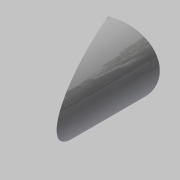
# Autodesk Inventor part: A1-19037-200-01 Trunk shell
Saved by Autodesk Inventor 2017.3 (Build 213257000, 257)
## iProperties
Created: 2019-08-22
Part Number: A1-19037-200-01 Trunk shell
Material: Steel, Mild
Document SubType Name: Sheet Metal
Designer: GVD
Density: 7.85 g/cm^3
Appearance: Steel
Project: A1-19037--CNUL Albian CST laterals
Mass: 348967 g
Surface Area: 25371.3 cm^2
Volume: 44454.4 cm^3
Description: 112 5/16" x 68 15/32" x 1 1/2" PLATE, A516 Gr.70N, ROLLED TO 37 1/4" OD
Flat Pattern Width: 131.612 cm
Flat Pattern Length: 134.186 cm
Flat Pattern Area: 17660.5 cm^2
Sheet Metal Rule: Default
Sheet Metal Width: 51.816 in
Sheet Metal Length: 52.829 in
Sheet Metal Area: 2737.386 in^2
Constructed By: Graeme_Van_Dongen
Project Name: CST laterals
Author: GVD
Autodesk Inventor part; units mm, degrees
ref_plane "YZ Plane" through (0, 0, 0) normal (1, 0, 0) x (0, 1, 0)
ref_plane "XZ Plane" through (0, 0, 0) normal (0, 1, 0) x (-1, 0, 0)
ref_plane "XY Plane" through (0, 0, 0) normal (0, 0, 1) x (1, 0, 0)
sketch "Sketch1" plane through (0, 0, 0) normal (0, 0, 1) x (1, 0, 0)
  circle A0 centre (0, 0) radius 434.975
  circle A1 centre (0, 0) radius 473.075
  circle A2 centre (0, 0) radius 436.5625
  dimension "d0" = 869.95
  dimension "d1" = 946.15
  dimension "d10" = 873.125
  constraints: 3 centre point, 3 coincident
  measures "d0" diameter of A0
  measures "d1" diameter of A1
  measures "d10" diameter of A2
extrude "Extrusion1" add sketch "Sketch1" along normal blind 1294.4 and the other way blind 444.4 contours A1 | A2
sketch "Sketch2" plane through (0, 0, 0) normal (0, 1, 0) x (-1, 0, 0)
  line L0 (0, 0) -> (-473.075, 1142.1041)
  line L1 (-473.075, -444.4) -> (-473.075, 1294.4) projected
  line L2 (-473.075, 1142.1041) -> (-473.075, -195.9541)
  line L3 (-473.075, -444.4) -> (-473.075, 1294.4) projected
  line L4 (0, 0) -> (-473.075, -195.9541)
  dimension "d79" = 22.5
  constraints: 6 end point, 2 point on line, 1 coincident, 1 perpendicular
  measures "d79" angle of L1 L0
extrude "Extrusion2" cut sketch "Sketch2" along normal through all both and the other way through all keep common part
equation "\"BendRadius\" = Thickness"
equation "\"BendReliefWidth\" = Thickness"
equation "\"BendReliefDepth\" = 0.5 * Thickness"
equation "\"CornerReliefSize\" = 4 * Thickness"
equation "\"MinimumRemnant\" = 2 * Thickness"
equation "\"TransitionRadius\" = BendRadius"
equation "\"JacobiRadiusSize\" = Thickness"
equation "\"GapSize\" = Thickness"
equation "\"Thickness\" = 38.1"
body "Solid1"
